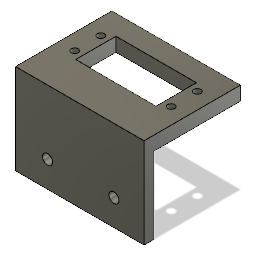
motor case v3 (Autodesk Fusion 360 design; units mm, degrees)
Autodesk Fusion 360 part; units mm, degrees
sketch "Sketch1" plane through (0, 0, 0) normal (0, 1, 0) x (1, 0, 0)
sketch "Sketch2" plane through (0, 0, 0) normal (0, 1, 0) x (1, 0, 0)
  line L0 (0, 0) -> (40, 0)
  line L1 (40, 0) -> (40, 20)
  line L2 (40, 20) -> (0, 20)
  line L3 (0, 20) -> (0, 0)
  line L4 (-12, -18) -> (52, -18)
  line L5 (52, -18) -> (52, 30)
  line L6 (52, 30) -> (-12, 30)
  line L7 (-12, 30) -> (-12, -18)
  line L8 (44, 20) -> (44, 16.5) construction
  line L9 (44, 0) -> (44, 3.5) construction
  line L10 (40, 16.5) -> (44, 16.5) construction
  line L11 (40, 3.5) -> (44, 3.5) construction
  circle A0 centre (44, 16.5) radius 1.75
  circle A1 centre (44, 3.5) radius 1.75
  line L12 (-4, 20) -> (-4, 16.5) construction
  line L13 (0, 16.5) -> (-4, 16.5) construction
  line L14 (0, 3.5142) -> (-4, 3.5126) construction
  line L15 (-4, 0.0126) -> (-4, 3.5126) construction
  circle A2 centre (-4, 16.5) radius 1.75
  circle A3 centre (-4, 3.5126) radius 1.75
  dimension "d1" = 40
  dimension "d2" = 20
  dimension "d8" = 18
  dimension "d9" = 10
  dimension "d10" = 3.5
  dimension "d11" = 3.5
  dimension "d12" = 4
  dimension "d13" = 4
  dimension "d14" = 3.5
  dimension "d15" = 3.5
  dimension "d16" = 3.5
  dimension "d17" = 4
  dimension "d18" = 4
  dimension "d19" = 3.5
  dimension "d20" = 3.5
  dimension "d21" = 3.5
  dimension "d22" = 12
  dimension "d23" = 12
  measures "d1" distance of L0.start L0.end
  measures "d2" distance of L0.start L2.end
  measures "d8" distance of L0 L4
  measures "d9" distance of L2 L6
  measures "d10" distance of L8.start L8.end
  measures "d11" distance of L9.start L9.end
  measures "d12" distance of L10.start L8.end
  measures "d13" distance of L11.start L9.end
  measures "d14" diameter of A0
  measures "d15" diameter of A1
  measures "d16" distance of L12.start L12.end
  measures "d17" distance of L13.start L12.end
  measures "d18" distance of L14.start L14.end
  measures "d19" distance of L15.start L14.end
  measures "d20" diameter of A2
  measures "d21" diameter of A3
  measures "d22" distance of L3 L7
  measures "d23" distance of L1 L5
extrude "Extrude1" add sketch "Sketch2" along normal blind 7
sketch "Sketch3" plane through (0, 7, 0) normal (0, 1, 0) x (-1, 0, 0)
  circle A0 centre (4, -3.5126) radius 1.75
  circle A1 centre (-44, -16.5) radius 1.75
  circle A2 centre (4, -16.5) radius 1.75
  circle A3 centre (-44, -3.5) radius 1.75
  line L0 (0, 0) -> (0, -20)
  line L1 (0, -20) -> (-40, -20)
  line L2 (-40, -20) -> (-40, 0)
  line L3 (-40, 0) -> (0, 0)
  line L4 (12, -30) -> (12, 18)
  line L5 (12, 18) -> (-52, 18)
  line L6 (-52, 18) -> (-52, -30)
  line L7 (-52, -30) -> (12, -30)
  line L8 (12, 18) -> (-52, 18)
  line L9 (-52, 18) -> (-52, 13)
  line L10 (-52, 13) -> (12, 13)
  line L11 (12, 13) -> (12, 18)
  dimension "d26" = 5
  measures "d26" distance of L4.end L10.end
extrude "Extrude2" add sketch "Sketch3" against normal blind 45 contours L4 L5 L6 L8 L9 L10 L11
sketch "Sketch4" plane through (0, 0, 13) normal (0, 0, -1) x (-1, 0, 0)
  line L0 (12, 0) -> (-52, 0)
  line L1 (-52, 0) -> (-52, -38)
  line L2 (-52, -38) -> (12, -38)
  line L3 (12, -38) -> (12, 0)
  circle A0 centre (-37, -25) radius 2.5
  circle A1 centre (-4, -25) radius 2.5
  dimension "d29" = 5
  dimension "d30" = 5
  measures "d29" diameter of A0
  measures "d30" diameter of A1
extrude "Extrude3" cut sketch "Sketch4" against normal blind 10 contours A0 | A1
